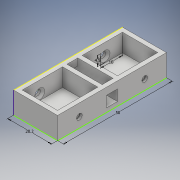
# Autodesk Inventor part: digit_holder_C
Saved by Autodesk Inventor 2018 (Build 220112000, 112)
## iProperties
Created: 2021-04-22
Part Number: digit_holder_C
Material: Generic
Document SubType Name: Modeling
Designer: Kevin
Density: 1 g/cm^3
Appearance: Default
Author: Kevin
Autodesk Inventor part; units mm, degrees
ref_plane "YZ Plane" through (0, 0, 0) normal (1, 0, 0) x (0, 1, 0)
ref_plane "XZ Plane" through (0, 0, 0) normal (0, 1, 0) x (-1, 0, 0)
ref_plane "XY Plane" through (0, 0, 0) normal (0, 0, 1) x (1, 0, 0)
sketch "Sketch3" plane through (0, 0, 0) normal (0, 0, 1) x (1, 0, 0)
  line L0 (-10.1, 25) -> (10.1, 25)
  line L1 (10.1, 25) -> (10.1, -25)
  line L2 (10.1, -25) -> (-10.1, -25)
  line L3 (-10.1, -25) -> (-10.1, 25)
  point P0 (0, 0)
  dimension "d26" = 20.2
  dimension "d27" = 50
  constraints: 8 end point, 2 parallel, 1 horizontal, 1 perpendicular
  measures "d26" distance of L1.end L2.end
  measures "d27" distance of L0.end L1.end
extrude "Extrusion3" add sketch "Sketch3" along normal blind 1.8
sketch "Sketch4" plane through (0, 0, 1.8) normal (0, 0, 1) x (1, 0, 0)
  line L0 (-8.1, 23) -> (8.1, 23)
  line L1 (8.1, -23) -> (-8.1, -23)
  line L2 (-8.1, 0) -> (-8.1, 2.5)
  line L3 (-8.1, 2.5) -> (8.1, 2.5)
  line L4 (8.1, 4.5) -> (-8.1, 4.5)
  line L5 (-8.1, 0) -> (-8.1, -2.5)
  line L6 (-8.1, -2.5) -> (8.1, -2.5)
  line L7 (8.1, -4.5) -> (-8.1, -4.5)
  line L8 (-8.1, 4.5) -> (-8.1, 23)
  line L9 (8.1, 23) -> (8.1, 4.5)
  line L10 (8.1, 2.5) -> (8.1, -2.5)
  line L11 (8.1, -4.5) -> (8.1, -23)
  line L12 (-10.1, 25) -> (-10.1, -25) projected
  line L13 (10.1, -25) -> (10.1, 25) projected
  line L14 (-10.1, 25) -> (10.1, 25)
  line L15 (10.1, 25) -> (10.1, -25)
  line L16 (10.1, -25) -> (-10.1, -25)
  line L17 (-10.1, -25) -> (-10.1, 25)
  line L18 (-8.1, -23) -> (-8.1, -4.5)
  line L19 (-8.1, -2.5) -> (-8.1, 2.5)
  point P0 (0, 0)
  dimension "d39" = 2.5
  dimension "d40" = 2.5
  dimension "d44" = 2
  dimension "d45" = 2
  dimension "d48" = 2
  dimension "d49" = 2
  dimension "d50" = 2
  dimension "d51" = 2
  dimension "d52" = 2
  dimension "d53" = 2
  dimension "d56" = 2
  dimension "d57" = 2
  constraints: 36 end point, 14 parallel, 4 horizontal, 4 perpendicular, 1 midpoint
  measures "d39" distance from line of point (0, 0) L3
  measures "d40" distance from line of point (0, 0) L6
  measures "d44" distance between parallel lines of L3 L4
  measures "d45" distance between parallel lines of L7 L6
  measures "d48" distance between parallel lines of L14 L0
  measures "d49" distance between parallel lines of L12 L8
  measures "d50" distance between parallel lines of L13 L9
  measures "d51" distance between parallel lines of L17 L18
  measures "d52" distance between parallel lines of L13 L11
  measures "d53" distance between parallel lines of L16 L1
  measures "d56" distance between parallel lines of L12 L2
  measures "d57" distance between parallel lines of L15 L10
extrude "Extrusion4" add sketch "Sketch4" along normal blind 8.2
sketch "Sketch5" plane through (10.1, -25, 0) normal (1, 0, 0) x (0, 0, -1)
  line L0 (-1.8, 27.5) -> (-10, 27.5) projected
  line L1 (-1.8, 22.5) -> (-10, 22.5) projected
  line L2 (-10, 27.5) -> (-1.8, 27.5)
  line L3 (-1.8, 27.5) -> (-1.8, 22.5)
  line L4 (-1.8, 22.5) -> (-10, 22.5)
  line L5 (-10, 22.5) -> (-10, 27.5)
  point P0 (0, 25)
  constraints: 8 end point, 2 parallel, 1 horizontal, 1 perpendicular
extrude "Extrusion5" cut sketch "Sketch5" against normal blind 8.2
sketch "Sketch6" plane through (-10.1, -25, 0) normal (-1, 0, 0) x (0, 0, 1)
  line L0 (1.8, 27.5) -> (1.8, 22.5) projected
  line L1 (1.8, 22.5) -> (6.8, 22.5)
  line L2 (6.8, 22.5) -> (6.8, 27.5)
  line L3 (6.8, 27.5) -> (1.8, 27.5)
  line L4 (1.8, 27.5) -> (1.8, 22.5)
  point P0 (0, 25)
  dimension "d60" = 5
  dimension "d61" = 5
  constraints: 8 end point, 2 parallel, 1 horizontal, 1 perpendicular
  measures "d60" distance of L3.end L2.end
  measures "d61" distance of L2.end L1.end
extrude "Extrusion6" cut sketch "Sketch6" against normal blind 8.2
sketch "Sketch7" plane through (-10.1, -25, 0) normal (-1, 0, 0) x (0, 0, 1)
  line L0 (0, 50) -> (10, 50) projected
  line L1 (0, 0) -> (0, 50) projected
  line L2 (0, 0) -> (10, 0)
  line L3 (10, 50) -> (10, 0) projected
  line L4 (10, 29.5) -> (10, 48) projected
  line L5 (10, 20.5) -> (10, 2) projected
  point P0 (0, 25)
  point P1 (4.5, 40)
  point P2 (4.5, 10)
  dimension "d66" = 10
  dimension "d67" = 4.5
  constraints: 2 end point
  measures "d66" distance from line of L0 point (4.5, 40)
  measures "d67" distance from line of L1 point (4.5, 40)
hole "Hole1" at (-10.1, 15, 4.5) at (-10.1, -15, 4.5) direction (1, 0, 0) diameter 2.6 depth 2 tip angle 118
chamfer "Chamfer3" distance 1 angle 45 2 edges at (-8.1, -15, 3.2) (-8.1, 15, 3.2)
sketch "Sketch10" plane through (10.1, -25, 0) normal (1, 0, 0) x (0, 0, -1)
  circle A0 centre (-4.5, 40) radius 2.3 projected
  circle A1 centre (-4.5, 10) radius 2.3 projected
  point P0 (0, 25)
  constraints: 3 coincident
hole "Hole6" at (10.1, -15, 4.5) at (10.1, 15, 4.5) direction (-1, 0, 0) diameter 2.6 depth 2 tip angle 118
sketch "Sketch11" plane through (-10.1, 2.5, 1.8) normal (0, -1, 0) x (1, 0, 0)
  line L0 (2, 8.2) -> (20.2, 8.2) projected
  line L1 (20.2, 8.2) -> (18.2, 8.2)
  line L2 (18.2, 8.2) -> (18.2, 5)
  line L3 (18.2, 5) -> (20.2, 5)
  line L4 (20.2, 5) -> (20.2, 8.2)
  point P0 (10.1, -1.8)
  dimension "d141" = 2
  dimension "d142" = 3.2
  constraints: 8 end point, 2 parallel, 1 horizontal, 1 perpendicular
  measures "d141" distance of L3.end L2.end
  measures "d142" distance of L2.end L1.end
extrude "Extrusion9" add sketch "Sketch11" along normal blind 10
chamfer "Chamfer4" distance 1 angle 45 2 edges at (8.1, 15, 5.8) (8.1, -15, 5.8)
body "Solid2"
